Laminated stator (Autodesk Fusion 360 design; units mm, degrees)
Autodesk Fusion 360 part; units mm, degrees
sketch "Esquisse1" plane through (0, 0, 0) normal (0, 0, 1) x (1, 0, 0)
  circle A0 centre (0, 0) radius 8.5
  line L0 (1.25, 10.1502) -> (1.25, 17.6106)
  arc A1 (1.25, 10.1502) -> (1.665, 9.6575) centre (1.75, 10.1502) ccw
  arc A2 (4.0366, 19.8946) -> (-0.0106, 20.3) centre (0, 0) ccw
  arc A3 (3.3867, 9.1962) -> (1.665, 9.6575) centre (0, 0) ccw
  arc A4 (3.3154, 19) -> (1.25, 17.6106) centre (2.75, 17.6106) ccw
  arc A5 (3.3154, 19) -> (4.0366, 19.8946) centre (3.5415, 19.5558) ccw
  line L1 (-1.25, 10.1502) -> (-1.25, 17.6093)
  arc A6 (-1.6651, 9.6575) -> (-1.25, 10.1502) centre (-1.75, 10.1502) ccw
  arc A7 (-1.25, 17.6093) -> (-3.3147, 19.0003) centre (-2.75, 17.6106) ccw
  arc A8 (-4.0366, 19.8946) -> (-3.3147, 19.0003) centre (-3.5415, 19.5558) ccw
  arc A9 (-0.0106, 20.3) -> (-4.0366, 19.8946) centre (0, 0) ccw
  arc A10 (-6.2708, 7.5311) -> (-6.1577, 8.1654) centre (-6.5907, 7.9154) ccw
  arc A11 (-10.1592, 17.575) -> (-13.4431, 15.2109) centre (0, 0) ccw
  arc A12 (-6.6288, 18.1122) -> (-7.7228, 15.8762) centre (-6.4237, 16.6262) ccw
  line L2 (-6.1577, 8.1654) -> (-9.8872, 14.6251)
  arc A13 (-6.6288, 18.1122) -> (-6.4515, 19.2476) centre (-6.7108, 18.7065) ccw
  arc A14 (-13.4431, 15.2109) -> (-12.3707, 14.7974) centre (-12.8449, 15.165) ccw
  arc A15 (-6.4515, 19.2476) -> (-10.1592, 17.575) centre (0, 0) ccw
  arc A16 (-9.8872, 14.6251) -> (-12.3707, 14.7974) centre (-11.1869, 13.8762) ccw
  arc A17 (-3.9926, 9.4154) -> (-3.3868, 9.1962) centre (-3.5596, 9.6654) ccw
  line L3 (-3.9926, 9.4154) -> (-7.7228, 15.8762)
  arc A18 (-9.1962, 3.3867) -> (-9.4154, 3.9926) centre (-9.6654, 3.5596) ccw
  arc A19 (-17.5856, 10.1408) -> (-19.2476, 6.4515) centre (0, 0) ccw
  arc A20 (-14.7968, 12.3712) -> (-14.6262, 9.8878) centre (-13.8762, 11.1869) ccw
  line L4 (-9.4154, 3.9926) -> (-15.8751, 7.7221)
  arc A21 (-14.7968, 12.3712) -> (-15.2109, 13.4431) centre (-15.165, 12.8449) ccw
  arc A22 (-19.2476, 6.4515) -> (-18.1121, 6.6295) centre (-18.7065, 6.7108) ccw
  arc A23 (-15.2109, 13.4431) -> (-17.5856, 10.1408) centre (0, 0) ccw
  arc A24 (-15.8751, 7.7221) -> (-18.1121, 6.6295) centre (-16.6262, 6.4237) ccw
  arc A25 (-8.1654, 6.1577) -> (-7.5311, 6.2707) centre (-7.9154, 6.5907) ccw
  line L5 (-8.1654, 6.1577) -> (-14.6262, 9.8878)
  arc A26 (-9.6575, -1.6651) -> (-10.1502, -1.25) centre (-10.1502, -1.75) ccw
  arc A27 (-20.3, -0.0106) -> (-19.8946, -4.0366) centre (0, 0) ccw
  arc A28 (-19, 3.3154) -> (-17.6106, 1.25) centre (-17.6106, 2.75) ccw
  line L6 (-10.1502, -1.25) -> (-17.6093, -1.25)
  arc A29 (-19, 3.3154) -> (-19.8946, 4.0366) centre (-19.5558, 3.5415) ccw
  arc A30 (-19.8946, -4.0366) -> (-19.0003, -3.3147) centre (-19.5558, -3.5415) ccw
  arc A31 (-19.8946, 4.0366) -> (-20.3, -0.0106) centre (0, 0) ccw
  arc A32 (-17.6093, -1.25) -> (-19.0003, -3.3147) centre (-17.6106, -2.75) ccw
  arc A33 (-10.1502, 1.25) -> (-9.6575, 1.665) centre (-10.1502, 1.75) ccw
  line L7 (-10.1502, 1.25) -> (-17.6106, 1.25)
  arc A34 (-7.5311, -6.2708) -> (-8.1654, -6.1577) centre (-7.9154, -6.5907) ccw
  arc A35 (-17.575, -10.1592) -> (-15.2109, -13.4431) centre (0, 0) ccw
  arc A36 (-18.1122, -6.6288) -> (-15.8762, -7.7228) centre (-16.6262, -6.4237) ccw
  line L8 (-8.1654, -6.1577) -> (-14.6251, -9.8872)
  arc A37 (-18.1122, -6.6288) -> (-19.2476, -6.4515) centre (-18.7065, -6.7108) ccw
  arc A38 (-15.2109, -13.4431) -> (-14.7974, -12.3707) centre (-15.165, -12.8449) ccw
  arc A39 (-19.2476, -6.4515) -> (-17.575, -10.1592) centre (0, 0) ccw
  arc A40 (-14.6251, -9.8872) -> (-14.7974, -12.3707) centre (-13.8762, -11.1869) ccw
  arc A41 (-9.4154, -3.9926) -> (-9.1962, -3.3868) centre (-9.6654, -3.5596) ccw
  line L9 (-9.4154, -3.9926) -> (-15.8762, -7.7228)
  arc A42 (-3.3867, -9.1962) -> (-3.9926, -9.4154) centre (-3.5596, -9.6654) ccw
  arc A43 (-10.1408, -17.5856) -> (-6.4515, -19.2476) centre (0, 0) ccw
  arc A44 (-12.3712, -14.7968) -> (-9.8878, -14.6262) centre (-11.1869, -13.8762) ccw
  line L10 (-3.9926, -9.4154) -> (-7.7221, -15.8751)
  arc A45 (-12.3712, -14.7968) -> (-13.4431, -15.2109) centre (-12.8449, -15.165) ccw
  arc A46 (-6.4515, -19.2476) -> (-6.6295, -18.1121) centre (-6.7108, -18.7065) ccw
  arc A47 (-13.4431, -15.2109) -> (-10.1408, -17.5856) centre (0, 0) ccw
  arc A48 (-7.7221, -15.8751) -> (-6.6295, -18.1121) centre (-6.4237, -16.6262) ccw
  arc A49 (-6.1577, -8.1654) -> (-6.2707, -7.5311) centre (-6.5907, -7.9154) ccw
  line L11 (-6.1577, -8.1654) -> (-9.8878, -14.6262)
  arc A50 (1.6651, -9.6575) -> (1.25, -10.1502) centre (1.75, -10.1502) ccw
  arc A51 (0.0106, -20.3) -> (4.0366, -19.8946) centre (0, 0) ccw
  arc A52 (-3.3154, -19) -> (-1.25, -17.6106) centre (-2.75, -17.6106) ccw
  line L12 (1.25, -10.1502) -> (1.25, -17.6093)
  arc A53 (-3.3154, -19) -> (-4.0366, -19.8946) centre (-3.5415, -19.5558) ccw
  arc A54 (4.0366, -19.8946) -> (3.3147, -19.0003) centre (3.5415, -19.5558) ccw
  arc A55 (-4.0366, -19.8946) -> (0.0106, -20.3) centre (0, 0) ccw
  arc A56 (1.25, -17.6093) -> (3.3147, -19.0003) centre (2.75, -17.6106) ccw
  arc A57 (-1.25, -10.1502) -> (-1.665, -9.6575) centre (-1.75, -10.1502) ccw
  line L13 (-1.25, -10.1502) -> (-1.25, -17.6106)
  arc A58 (6.2708, -7.5311) -> (6.1577, -8.1654) centre (6.5907, -7.9154) ccw
  arc A59 (10.1592, -17.575) -> (13.4431, -15.2109) centre (0, 0) ccw
  arc A60 (6.6288, -18.1122) -> (7.7228, -15.8762) centre (6.4237, -16.6262) ccw
  line L14 (6.1577, -8.1654) -> (9.8872, -14.6251)
  arc A61 (6.6288, -18.1122) -> (6.4515, -19.2476) centre (6.7108, -18.7065) ccw
  arc A62 (13.4431, -15.2109) -> (12.3707, -14.7974) centre (12.8449, -15.165) ccw
  arc A63 (6.4515, -19.2476) -> (10.1592, -17.575) centre (0, 0) ccw
  arc A64 (9.8872, -14.6251) -> (12.3707, -14.7974) centre (11.1869, -13.8762) ccw
  arc A65 (3.9926, -9.4154) -> (3.3868, -9.1962) centre (3.5596, -9.6654) ccw
  line L15 (3.9926, -9.4154) -> (7.7228, -15.8762)
  arc A66 (9.1962, -3.3867) -> (9.4154, -3.9926) centre (9.6654, -3.5596) ccw
  arc A67 (17.5856, -10.1408) -> (19.2476, -6.4515) centre (0, 0) ccw
  arc A68 (14.7968, -12.3712) -> (14.6262, -9.8878) centre (13.8762, -11.1869) ccw
  line L16 (9.4154, -3.9926) -> (15.8751, -7.7221)
  arc A69 (14.7968, -12.3712) -> (15.2109, -13.4431) centre (15.165, -12.8449) ccw
  arc A70 (19.2476, -6.4515) -> (18.1121, -6.6295) centre (18.7065, -6.7108) ccw
  arc A71 (15.2109, -13.4431) -> (17.5856, -10.1408) centre (0, 0) ccw
  arc A72 (15.8751, -7.7221) -> (18.1121, -6.6295) centre (16.6262, -6.4237) ccw
  arc A73 (8.1654, -6.1577) -> (7.5311, -6.2707) centre (7.9154, -6.5907) ccw
  line L17 (8.1654, -6.1577) -> (14.6262, -9.8878)
  arc A74 (9.6575, 1.6651) -> (10.1502, 1.25) centre (10.1502, 1.75) ccw
  arc A75 (20.3, 0.0106) -> (19.8946, 4.0366) centre (0, 0) ccw
  arc A76 (19, -3.3154) -> (17.6106, -1.25) centre (17.6106, -2.75) ccw
  line L18 (10.1502, 1.25) -> (17.6093, 1.25)
  arc A77 (19, -3.3154) -> (19.8946, -4.0366) centre (19.5558, -3.5415) ccw
  arc A78 (19.8946, 4.0366) -> (19.0003, 3.3147) centre (19.5558, 3.5415) ccw
  arc A79 (19.8946, -4.0366) -> (20.3, 0.0106) centre (0, 0) ccw
  arc A80 (17.6093, 1.25) -> (19.0003, 3.3147) centre (17.6106, 2.75) ccw
  arc A81 (10.1502, -1.25) -> (9.6575, -1.665) centre (10.1502, -1.75) ccw
  line L19 (10.1502, -1.25) -> (17.6106, -1.25)
  arc A82 (7.5311, 6.2708) -> (8.1654, 6.1577) centre (7.9154, 6.5907) ccw
  arc A83 (17.575, 10.1592) -> (15.2109, 13.4431) centre (0, 0) ccw
  arc A84 (18.1122, 6.6288) -> (15.8762, 7.7228) centre (16.6262, 6.4237) ccw
  line L20 (8.1654, 6.1577) -> (14.6251, 9.8872)
  arc A85 (18.1122, 6.6288) -> (19.2476, 6.4515) centre (18.7065, 6.7108) ccw
  arc A86 (15.2109, 13.4431) -> (14.7974, 12.3707) centre (15.165, 12.8449) ccw
  arc A87 (19.2476, 6.4515) -> (17.575, 10.1592) centre (0, 0) ccw
  arc A88 (14.6251, 9.8872) -> (14.7974, 12.3707) centre (13.8762, 11.1869) ccw
  arc A89 (9.4154, 3.9926) -> (9.1962, 3.3868) centre (9.6654, 3.5596) ccw
  line L21 (9.4154, 3.9926) -> (15.8762, 7.7228)
  arc A90 (3.3867, 9.1962) -> (3.9926, 9.4154) centre (3.5596, 9.6654) ccw
  arc A91 (10.1408, 17.5856) -> (6.4515, 19.2476) centre (0, 0) ccw
  arc A92 (12.3712, 14.7968) -> (9.8878, 14.6262) centre (11.1869, 13.8762) ccw
  line L22 (3.9926, 9.4154) -> (7.7221, 15.8751)
  arc A93 (12.3712, 14.7968) -> (13.4431, 15.2109) centre (12.8449, 15.165) ccw
  arc A94 (6.4515, 19.2476) -> (6.6295, 18.1121) centre (6.7108, 18.7065) ccw
  arc A95 (13.4431, 15.2109) -> (10.1408, 17.5856) centre (0, 0) ccw
  arc A96 (7.7221, 15.8751) -> (6.6295, 18.1121) centre (6.4237, 16.6262) ccw
  arc A97 (6.1577, 8.1654) -> (6.2707, 7.5311) centre (6.5907, 7.9154) ccw
  line L23 (6.1577, 8.1654) -> (9.8878, 14.6262)
  arc A98 (-1.6651, 9.6575) -> (-3.3868, 9.1962) centre (0, 0) ccw
  arc A99 (-6.2708, 7.5311) -> (-7.5311, 6.2707) centre (0, 0) ccw
  arc A100 (-9.1962, 3.3867) -> (-9.6575, 1.665) centre (0, 0) ccw
  arc A101 (-9.6575, -1.6651) -> (-9.1962, -3.3868) centre (0, 0) ccw
  arc A102 (-7.5311, -6.2708) -> (-6.2707, -7.5311) centre (0, 0) ccw
  arc A103 (-3.3867, -9.1962) -> (-1.665, -9.6575) centre (0, 0) ccw
  arc A104 (1.6651, -9.6575) -> (3.3868, -9.1962) centre (0, 0) ccw
  arc A105 (6.2708, -7.5311) -> (7.5311, -6.2707) centre (0, 0) ccw
  arc A106 (9.1962, -3.3867) -> (9.6575, -1.665) centre (0, 0) ccw
  arc A107 (9.6575, 1.6651) -> (9.1962, 3.3868) centre (0, 0) ccw
  arc A108 (7.5311, 6.2708) -> (6.2707, 7.5311) centre (0, 0) ccw
  point P0 (-1.6651, 9.6575)
  point P1 (-6.2708, 7.5311)
  point P2 (-9.1962, 3.3867)
  point P3 (-9.6575, -1.6651)
  point P4 (-7.5311, -6.2708)
  point P5 (-3.3867, -9.1962)
  point P6 (1.6651, -9.6575)
  point P7 (6.2708, -7.5311)
  point P8 (9.1962, -3.3867)
  point P9 (9.6575, 1.6651)
  point P10 (7.5311, 6.2708)
  dimension "d2" = 17
  dimension "d18" = 20.3
  dimension "d26" = 0.5
  dimension "d45" = 19
  dimension "d46" = 1.5
  dimension "d47" = 0.6
  dimension "d48" = 9.8
  dimension "d50" = 360
  dimension "d55" = 2.5
  dimension "d57" = 360
  constraint coincident A0.centre A2.centre
  constraint vertical L0
  constraint tangent L0 A1
  constraint tangent A1 A3
  constraint tangent A4 A5
  constraint tangent L0 A4
  constraint coincident A3.start A90.start
  constraint coincident A11.start A15.end
  measures "d2" diameter of A0
  measures "d18" radius of A2
  measures "d26" radius of A1
  measures "d45" vertical distance of A0.centre A4.start
  measures "d46" radius of A4
  measures "d47" radius of A5
  measures "d48" radius of A3
  measures "d55" distance of A8.start A13.end
extrude "Extrusion1" add sketch "Esquisse1" along normal blind 30
extrude "Extrusion1'" [suppressed]
copy_body "CutPasteBodies1" [suppressed]
